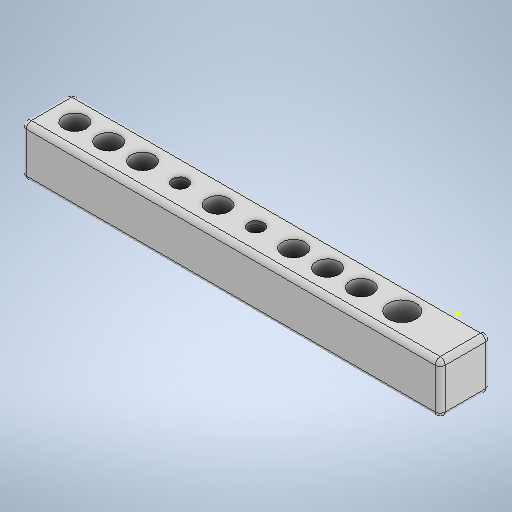
# Autodesk Inventor part: brazo de servo el d vdd - camara
Saved by Autodesk Inventor 2025.2 (Build 292293000, 293)
## iProperties
Created: 2025-03-30
Part Number: brazo de servo el d vdd - camara
Material: Generic
Document SubType Name: Modeling
Designer: maqmat
Density: 1 g/cm^3
Appearance: Default
Author: maqmat
Autodesk Inventor part; units mm, degrees
ref_plane "YZ Plane" through (0, 0, 0) normal (1, 0, 0) x (0, 1, 0)
ref_plane "XZ Plane" through (0, 0, 0) normal (0, 1, 0) x (-1, 0, 0)
ref_plane "XY Plane" through (0, 0, 0) normal (0, 0, 1) x (1, 0, 0)
sketch "Sketch1" plane through (0, 0, 0) normal (0, 1, 0) x (-1, 0, 0)
  line L0 (0, 0) -> (170, 0)
  line L1 (170, 0) -> (170, 10)
  line L2 (170, 10) -> (0, 10)
  line L3 (0, 10) -> (0, 0)
  dimension "d0" = 170
  dimension "d1" = 10
  constraints: 8 end point, 2 parallel, 1 horizontal, 1 perpendicular
  measures "d0" distance of L2.end L1.end
  measures "d1" distance of L1.end L0.end
extrude "Extrusion1" add sketch "Sketch1" along normal blind 10
sketch "Sketch2" plane through (0, 10, 0) normal (0, 1, 0) x (1, 0, 0)
  line L0 (0, -10) -> (0, 0) projected
  line L1 (0, -5) -> (-2.2, -5)
  circle A0 centre (-6.1, -5) radius 3.9
  line L2 (0, 0) -> (-170, 0) projected
  line L3 (-170, -10) -> (0, -10) projected
  circle A1 centre (-75, -5) radius 1.5
  circle A2 centre (-95, -5) radius 1.5
  dimension "d4" = 2.2
  dimension "d8" = 3
  dimension "d9" = 3
  constraints: 2 centre point, 2 end point, 1 horizontal, 1 horizontal alignment, 1 midpoint, 2 other
  measures "d4" distance of L1.start L1.end
  measures "d8" diameter of A1
  measures "d9" diameter of A2
extrude "Extrusion2" cut sketch "Sketch2" against normal blind 10 contours A1
extrude "Extrusion3" cut sketch "Sketch2" against normal blind 10 contours A2
extrude "Extrusion4" cut sketch "Sketch2" against normal blind 10 contours A0
sketch "Sketch3" plane through (0, 10, 0) normal (0, 1, 0) x (1, 0, 0)
  line L0 (-170, 0) -> (-170, -10) projected
  line L1 (-170, -5) -> (-10, -5)
  circle A0 centre (-6.1, -5) radius 3.9 projected
  line L2 (-165.7, -5) -> (-163.45, -5)
  circle A1 centre (-163.45, -5) radius 2.25
  circle A2 centre (-153.45, -5) radius 2.25
  circle A3 centre (-143.45, -5) radius 2.25
  circle A4 centre (-133.45, -5) radius 2.25
  circle A5 centre (-123.45, -5) radius 2.25
  circle A6 centre (-113.45, -5) radius 2.25
  circle A7 centre (-103.45, -5) radius 2.25
  circle A8 centre (-95, -5) radius 1.5 projected
  line L3 (-93.5, -5) -> (-93.5, -7.9104)
  circle A9 centre (-75, -5) radius 1.5 projected
  line L4 (-76.5, -5) -> (-76.5, -7.25)
  line L5 (-93.5, -5) -> (-76.5, -5)
  line L6 (-85, -5) -> (-93.5, -5)
  line L7 (-85, -5) -> (-76.5, -5)
  circle A10 centre (-80.75, -5) radius 2.25
  circle A11 centre (-89.25, -5) radius 2.25
  line L8 (-10, -5) -> (-12, -5)
  line L9 (-10, -5) -> (-14.3, -5)
  line L10 (-14.3, -5) -> (-16.55, -5)
  circle A12 centre (-16.55, -5) radius 2.25
  circle A13 centre (-26.55, -5) radius 2.25
  circle A14 centre (-36.55, -5) radius 2.25
  circle A15 centre (-46.55, -5) radius 2.25
  circle A16 centre (-56.55, -5) radius 2.25
  circle A17 centre (-66.55, -5) radius 2.25
  point P0 (0, 0)
  point P1 (-155.7, -5)
  point P2 (-145.7, -5)
  point P3 (-135.7, -5)
  point P4 (-125.7, -5)
  point P5 (-115.7, -5)
  point P6 (-105.7, -5)
  point P7 (-24.3, -5)
  point P8 (-34.3, -5)
  point P9 (-44.3, -5)
  point P10 (-54.3, -5)
  point P11 (-64.3, -5)
  dimension "d20" = 10
  dimension "d32" = 10
  constraints: 38 horizontal alignment, 18 end point, 4 midpoint, 4 vertical, 3 horizontal, 2 centre point, 2 coincident, 39 other
  measures "d20" distance of point (-163.45, -5) point (-153.45, -5)
  measures "d32" distance of point (-16.55, -5) point (-26.55, -5)
extrude "Extrusion5" cut sketch "Sketch3" against normal blind 10 contours A1 L1 | L1 A1 | L1 A12 | L1 A12 | A2 L1 | L1 A2 | A3 L1 | L1 A3 | A4 L1 | L1 A4 | A5 L1 | L1 A5 | A6 L1 | L1 A6 | A7 L1 | L1 A7 | A11 L1 | L1 A11 | A10 L1 | L1 A10 | A17 L1 | L1 A17 | A16 L1 | L1 A16 | A15 L1 | L1 A15 | A14 L1 | L1 A14 | A13 L1 | L1 A13
thread "Thread1" size "M3x0.5" class "6H" standard "ANSI Metric M Profile" full length
thread "Thread2" size "M3x0.5" class "6H" standard "ANSI Metric M Profile" full length
sketch "Sketch4" plane through (0, 10, 0) normal (0, 1, 0) x (1, 0, 0)
  circle A0 centre (-16.55, -5) radius 2.25 projected
  circle A1 centre (-16.55, -5) radius 2.25
  point P0 (0, 0)
  constraints: 1 centre point, 1 coincident
extrude "Extrusion6" add sketch "Sketch4" against normal blind 10
sketch "Sketch5" plane through (0, 0, 10) normal (1, 0, 0) x (0, 0, -1)
  line L0 (10, 0) -> (0, 0) projected
  line L1 (0, 0) -> (0, 10) projected
  line L2 (10, 0) -> (0, 0)
  line L3 (0, 0) -> (0, 10)
  line L4 (0, 10) -> (10, 10)
  line L5 (10, 10) -> (10, 0)
  constraints: 8 end point, 2 parallel, 1 horizontal, 1 perpendicular
extrude "Extrusion7" add sketch "Sketch5" along normal blind 10
sketch "Sketch6" plane through (10, 0, 10) normal (1, 0, 0) x (0, 0, -1)
  line L0 (0, 0) -> (10, 0) projected
  line L1 (0, 10) -> (0, 0) projected
  line L2 (10, 0) -> (0, 0)
  line L3 (0, 0) -> (0, 10)
  line L4 (0, 10) -> (10, 10)
  line L5 (10, 10) -> (10, 0)
  constraints: 8 end point, 2 parallel, 1 horizontal, 1 perpendicular
extrude "Extrusion8" add sketch "Sketch6" along normal blind 10
sketch "Sketch7" plane through (0, 10, 0) normal (0, 1, 0) x (1, 0, 0)
  point P0 (0, 0)
fillet "Fillet3" radius 1 11 edges at (-75, 10, 10) (-75, 0, 10) (-75, 10, 0) (20, 5, 10) (20, 5, 0) (20, 0, 5) (-170, 10, 5) (-170, 5, 10) (-170, 5, 0) (-170, 0, 5) (-75, 0, 0)
fillet "Fillet4" radius 1 3 edges at (19.7071, 9.7071, 9.7071) (19.7071, 9.7071, 0.2929) (20, 10, 5)
sketch "Sketch8" plane through (19, 1, 0) normal (0, 0, -1) x (-1, 0, 0)
  point P0 (19, -1)
sketch "Sketch9" plane through (0, 10, 0) normal (0, 1, 0) x (1, 0, 0)
  circle A0 centre (-6.1, -5) radius 3.9 projected
  circle A1 centre (-6.1, -5) radius 2.5
  point P0 (0, 0)
  dimension "d53" = 5
  constraints: 1 centre point, 1 coincident
  measures "d53" diameter of A1
extrude "Extrusion9" add sketch "Sketch9" against normal blind 10
sketch "Sketch10" plane through (0, 10, 0) normal (0, 1, 0) x (1, 0, 0)
  circle A0 centre (-6.1, -5) radius 2.5 projected
  line L0 (-3.6, -5) -> (1.4, -5)
  line L1 (19, -9) -> (19, -1) projected
  line L2 (1.4, -5) -> (-76.5, -5)
  circle A1 centre (-75, -5) radius 1.5 projected
  line L3 (-76.5, -5) -> (-76.5, -10.0231)
  line L4 (-76.5, -10.0231) -> (-76.5, 0)
  line L5 (-76.5, -10.0231) -> (-169.9715, -10.0231)
  line L6 (-169, -9) -> (19, -9) projected
  line L7 (-169.9715, 0) -> (-76.5, 0)
  line L8 (-169.9715, -10.0231) -> (-170.1763, -9.372)
  line L9 (-170.1763, -9.372) -> (-170.4489, -3.7164)
  line L10 (-170.4489, -3.7164) -> (-170.4593, -3.5)
  line L11 (-170.4593, -3.5) -> (-170.4593, -0.543)
  line L12 (-170.4593, -0.543) -> (-169.9715, 0)
  point P0 (0, 0)
  dimension "d56" = 5
  constraints: 22 end point, 3 point on line, 3 vertical, 2 horizontal alignment, 1 parallel, 1 perpendicular, 2 other
  measures "d56" distance of L0.start L0.end
extrude "Extrusion10" cut sketch "Sketch10" against normal blind 10 contours L3 L5 L8 L9 L10 L11 L12 L7 L4
sketch "Sketch11" plane through (0, 10, 0) normal (0, 1, 0) x (1, 0, 0)
  circle A0 centre (-75, -5) radius 1.5 projected
  circle A1 centre (-75, -5) radius 1.5
  circle A2 centre (-66.55, -5) radius 2.25 projected
  circle A3 centre (-66.55, -5) radius 2.25
  circle A4 centre (-56.55, -5) radius 2.25 projected
  circle A5 centre (-56.55, -5) radius 2.25
  circle A6 centre (-46.55, -5) radius 2.25 projected
  circle A7 centre (-46.55, -5) radius 2.25
  circle A8 centre (-36.55, -5) radius 2.25 projected
  circle A9 centre (-36.55, -5) radius 2.25
  circle A10 centre (-26.55, -5) radius 2.25 projected
  circle A11 centre (-26.55, -5) radius 2.25
  point P0 (0, 0)
  point P1 (-76.5, -5)
  constraints: 6 centre point, 6 coincident, 1 horizontal alignment
extrude "Extrusion11" add sketch "Sketch11" against normal blind 10
sketch "Sketch12" plane through (0, 10, 0) normal (0, 1, 0) x (1, 0, 0)
  circle A0 centre (-6.1, -5) radius 2.5 projected
  line L0 (-8.6, -5) -> (-76.5, -5)
  line L1 (-76.5, -9) -> (-76.5, -1) projected
  line L2 (-42.55, -5) -> (-27.55, -5)
  line L3 (-42.55, -5) -> (-57.55, -5)
  line L4 (-42.55, -5) -> (-50.05, -5)
  line L5 (-42.55, -5) -> (-35.05, -5)
  circle A1 centre (-50.05, -5) radius 1.5
  circle A2 centre (-35.05, -5) radius 1.5
  line L6 (-3.6, -5) -> (6.4143, -5)
  line L7 (6.4143, -5) -> (6.4143, -10.3738)
  line L8 (6.4143, -10.3738) -> (6.4143, 1.3096)
  line L9 (6.4143, 1.3096) -> (23.7189, 1.3096)
  line L10 (23.7189, 1.3096) -> (24.3802, -13.5702)
  line L11 (24.3802, -13.5702) -> (6.4143, -10.3738)
  point P0 (0, 0)
  dimension "d61" = 15
  dimension "d62" = 15
  dimension "d63" = 3
  dimension "d64" = 3
  constraints: 22 end point, 4 midpoint, 3 point on line, 2 centre point, 2 coincident, 2 perpendicular, 2 point on circle, 1 horizontal
  measures "d61" distance of L2.start L2.end
  measures "d62" distance of L2.start L3.end
  measures "d63" diameter of A1
  measures "d64" diameter of A2
extrude "Extrusion12" cut sketch "Sketch12" against normal blind 10 contours A2 L0 | L0 A2 | A1 L0 | L0 A1 | L8 L9 L10 L11 L7
sketch "Sketch13" plane through (0, 10, 0) normal (0, 1, 0) x (1, 0, 0)
  circle A0 centre (-50.05, -5) radius 1.5 projected
  line L0 (-48.55, -5) -> (-36.55, -5)
  circle A1 centre (-35.05, -5) radius 1.5 projected
  circle A2 centre (-42.55, -5) radius 2.25
  line L1 (-51.55, -5) -> (-55.25, -5)
  line L2 (-33.55, -5) -> (-29.85, -5)
  circle A3 centre (-57.5, -5) radius 2.25
  circle A4 centre (-27.6, -5) radius 2.25
  circle A5 centre (-20.9, -5) radius 2.25
  circle A6 centre (-14.2, -5) radius 2.25
  circle A7 centre (-64.2, -5) radius 2.25
  circle A8 centre (-70.9, -5) radius 2.25
  point P0 (0, 0)
  dimension "d67" = 4.5
  dimension "d68" = 3.7
  dimension "d69" = 3.7
  dimension "d71" = 4.5
  dimension "d73" = 4.5
  dimension "d83" = 6.7
  dimension "d90" = 6.7
  constraints: 7 centre point, 6 end point, 4 point on circle, 4 point on line, 3 horizontal, 1 midpoint, 8 other
  measures "d67" diameter of A2
  measures "d68" distance of L1.start L1.end
  measures "d69" distance of L2.start L2.end
  measures "d71" diameter of A3
  measures "d73" diameter of A4
  measures "d83" distance of A4.centre A5.centre
  measures "d90" distance of A3.centre A7.centre
extrude "Extrusion13" cut sketch "Sketch13" against normal blind 10 contours A3 | A4 | A5 | A6 | A7 | A8
sketch "Sketch14" plane through (0, 10, 0) normal (0, 1, 0) x (1, 0, 0)
  circle A0 centre (-57.5, -5) radius 2.25 projected
  line L0 (-55.25, -5) -> (-29.85, -5)
  circle A1 centre (-27.6, -5) radius 2.25 projected
  circle A2 centre (-42.55, -5) radius 2.25
  point P0 (0, 0)
  dimension "d97" = 4.5
  constraints: 2 end point, 2 horizontal alignment, 1 centre point, 1 horizontal, 1 midpoint, 2 other
  measures "d97" diameter of A2
extrude "Extrusion14" cut sketch "Sketch14" against normal blind 10 contours A2 L0 | L0 A2
thread "Thread3" size "M3x0.5" class "6H" standard "ANSI Metric M Profile" full length
thread "Thread4" size "M3x0.5" class "6H" standard "ANSI Metric M Profile" full length
fillet "Fillet5" radius 1 16 edges at (-76.5, 9.7071, 9.7071) (-76.5, 5, 10) (-76.5, 0.2929, 9.7071) (-76.5, 0, 5) (-76.5, 0.2929, 0.2929) (-76.5, 5, 0) (-76.5, 9.7071, 0.2929) (-76.5, 10, 5) (6.4143, 9.7071, 0.2929) (6.4143, 5, 0) (6.4143, 0.2929, 0.2929) (6.4143, 0, 5) (6.4143, 0.2929, 9.7071) (6.4143, 5, 10) (6.4143, 9.7071, 9.7071) (6.4143, 10, 5)
sketch "Sketch15" plane through (0, 10, 0) normal (0, 1, 0) x (1, 0, 0)
  circle A0 centre (-6.1, -5) radius 2.5 projected
  circle A1 centre (-6.1, -5) radius 2.75
  point P0 (0, 0)
  dimension "d105" = 5.5
  constraints: 1 centre point, 1 coincident
  measures "d105" diameter of A1
extrude "Extrusion15" cut sketch "Sketch15" against normal blind 10 contours A0 | A1
body "Solid1"
